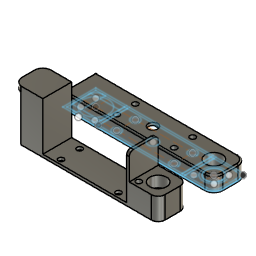
laserHolder v8 (Autodesk Fusion 360 design; units mm, degrees)
Autodesk Fusion 360 part; units mm, degrees
note: some values were not read from the file. Set by a fixed rule: which sketch regions a step uses.
sketch "Sketch1" plane through (0, 0, 0) normal (0, 0, 1) x (1, 0, 0)
  line L0 (0, 0) -> (61, 0)
  line L1 (61, 0) -> (61, 21)
  line L2 (61, 21) -> (0, 21)
  line L3 (0, 21) -> (0, 0)
  line L4 (61, 0) -> (63, 0)
  line L5 (63, 0) -> (63, 21)
  line L6 (63, 21) -> (61, 21)
  line L7 (61, 21) -> (61, 0)
  line L8 (0, 21) -> (-2, 21)
  line L9 (-2, 21) -> (-2, 0)
  line L10 (-2, 0) -> (0, 0)
  line L11 (0, 0) -> (0, 21)
  line L12 (-2, 21) -> (-23, 21)
  line L13 (-23, 21) -> (-23, 0)
  line L14 (-23, 0) -> (-2, 0)
  line L15 (-2, 0) -> (-2, 21)
  line L16 (-12.5, 21) -> (-12.5, -1.4858) construction
  line L17 (-23, 10.5) -> (-2, 10.5) construction
  circle A0 centre (-12.5, 10.5) radius 9.2
  line L18 (-23, 21) -> (-16, 21)
  line L19 (-16, 21) -> (-16, 0)
  line L20 (-16, 0) -> (-23, 0)
  line L21 (-23, 0) -> (-23, 21)
  line L22 (63, 21) -> (79, 21)
  line L23 (84, 16) -> (84, 5)
  line L24 (79, 0) -> (63, 0)
  line L25 (63, 0) -> (63, 21)
  line L26 (73.5, 21) -> (73.5, 0) construction
  line L27 (63, 10.5) -> (84, 10.5) construction
  circle A1 centre (73.5, 10.5) radius 5
  circle A2 centre (73.5, 10.5) radius 6.1
  arc A3 (84, 16) -> (79, 21) centre (79, 16) ccw
  arc A4 (79, 0) -> (84, 5) centre (79, 5) ccw
  circle A5 centre (-4.3879, 2.2553) radius 1.5
  circle A6 centre (66.1765, 3.7347) radius 2
  line L28 (0, 3.3) -> (61, 3.3) construction
  line L29 (0, 16.8) -> (61, 16.8) construction
  line L30 (10.02, 0) -> (10.02, 21) construction
  line L31 (51.78, 0) -> (51.78, 21) construction
  circle A7 centre (10.02, 3.3) radius 2
  circle A8 centre (51.78, 3.3) radius 2
  circle A9 centre (10.02, 16.8) radius 2
  circle A10 centre (51.78, 16.8) radius 2
  point P0 (84, 21)
  dimension "d1" = 61
  dimension "d2" = 21
  dimension "d3" = 2
  dimension "d4" = 2
  dimension "d5" = 21
  dimension "d6" = 21
  dimension "d7" = 21
  dimension "d8" = 18.4
  dimension "d9" = 7
  dimension "d10" = 21
  dimension "d11" = 21
  dimension "d12" = 21
  dimension "d13" = 10
  dimension "d14" = 12.2
  dimension "d15" = 5
  dimension "d35" = 3
  dimension "d38" = 4
  dimension "d44" = 3.3
  dimension "d45" = 9.22
  dimension "d46" = 41.76
  dimension "d47" = 13.5
  dimension "d48" = 4
  dimension "d49" = 4
  dimension "d50" = 4
  dimension "d51" = 4
  constraint horizontal L0
  constraint vertical L1
  constraint horizontal L2
  constraint vertical L3
  constraint coincident L0.start L3.end
  constraint horizontal L4
  constraint vertical L5
  constraint horizontal L6
  constraint vertical L7
  constraint horizontal L8
  constraint vertical L9
  constraint horizontal L10
  constraint vertical L11
  constraint horizontal L12
  constraint vertical L13
  constraint horizontal L14
  constraint vertical L15
  constraint midpoint L12 L16.start
  constraint perpendicular L14 L16
  constraint midpoint L13 L17.start
  constraint midpoint L9 L17.end
  constraint midpoint L17 A0.centre
  constraint horizontal L18
  constraint vertical L19
  constraint horizontal L20
  constraint vertical L21
  constraint horizontal L22
  constraint vertical L23
  constraint horizontal L24
  constraint vertical L25
  constraint midpoint L25 L27.start
  constraint midpoint L26 A1.centre
  constraint concentric A1 A2
  constraint coincident L22 L26.start
  constraint coincident L23 L27.end
  constraint coincident P0 L22
  constraint coincident P0 L23
  constraint tangent L22 A3
  constraint tangent L23 A3
  constraint coincident L24 L26.end
  constraint tangent L23 A4
  constraint tangent L24 A4
  constraint equal A3 A4
  constraint coincident L3 L28.start
  constraint perpendicular L3 L28
  constraint coincident L1 L28.end
  constraint coincident L3 L29.start
  constraint perpendicular L3 L29
  constraint coincident L7 L29.end
  constraint coincident L0 L30.start
  constraint coincident L2 L30.end
  constraint perpendicular L2 L30
  constraint coincident L0 L31.start
  constraint coincident L2 L31.end
  constraint perpendicular L2 L31
  constraint coincident L30 A7.centre
  constraint coincident L28 A7.centre
  constraint coincident L31 A8.centre
  constraint coincident L28 A8.centre
  constraint coincident L30 A9.centre
  constraint coincident L29 A9.centre
  constraint coincident L31 A10.centre
  constraint coincident L29 A10.centre
  measures "d1" distance of L0.start L0.end
  measures "d2" distance of L0.start L2.end
  measures "d3" distance of L0.end L4.end
  measures "d4" distance of L2.end L8.end
  measures "d5" distance of L2.end L0.start
  measures "d6" distance of L8.end L12.end
  measures "d7" distance of L8.end L9.end
  measures "d8" diameter of A0
  measures "d9" distance of L12.end L18.end
  measures "d10" distance of L12.end L13.end
  measures "d11" distance of L5.end P0
  measures "d12" distance of L5.end L4.end
  measures "d13" diameter of A1
  measures "d14" diameter of A2
  measures "d15" radius of A3
  measures "d35" diameter of A5
  measures "d38" diameter of A6
  measures "d44" distance of L0 L28
  measures "d45" distance of L1 L31
  measures "d46" distance of L30 L31
  measures "d47" distance of L28 L29
  measures "d48" diameter of A7
  measures "d49" diameter of A8
  measures "d50" diameter of A9
  measures "d51" diameter of A10
extrude "Extrude1" add sketch "Sketch1" along normal blind 2 contours L0 L1 L2 L3 L7 L11 | A7 | A8 | A9 | A10 makes body 1
extrude "Extrude2" add sketch "Sketch1" along normal blind 35 contours L3 L8 L9 L10 L11 L15 | L9 L12 L14 L15 A0 L19 | A5 bodies 1
extrude "Extrude3" add sketch "Sketch1" along normal blind 35 contours L1 L4 L5 L6 L7 L25 bodies 1
extrude "Extrude4" add sketch "Sketch1" along normal blind 16 contours L5 L22 L23 L24 L25 A3 A4 | A2 | A6 bodies 1
extrude "Extrude5" cut sketch "Sketch1" along normal blind 8 from surface at 8 contours A2 bodies 1
sketch "Sketch2" plane through (0, 0, 35) normal (0, 0, 1) x (-1, 0, 0)
  line L0 (16, -1.9918) -> (16, 0)
  line L1 (16, 0) -> (0, 0)
  line L2 (0, 0) -> (0, -21)
  line L3 (0, -21) -> (16, -21)
  line L4 (16, -21) -> (16, -19.0082)
  arc A0 (16, -1.9918) -> (16, -19.0082) centre (12.5, -10.5) ccw
  line L5 (0, 0) -> (15, 0)
  line L6 (21, -6) -> (21, -15)
  line L7 (15, -21) -> (0, -21)
  line L8 (0, -21) -> (0, 0)
  arc A1 (21, -6) -> (15, 0) centre (15, -6) ccw
  arc A2 (15, -21) -> (21, -15) centre (15, -15) ccw
  point P0 (21, 0)
  dimension "d27" = 21
  dimension "d28" = 21
  dimension "d29" = 6
  dimension "d30" = 6
  constraint horizontal L5
  constraint vertical L6
  constraint horizontal L7
  constraint vertical L8
  constraint coincident L1.end L2.start
  constraint coincident P0 L5
  constraint coincident P0 L6
  constraint tangent L5 A1
  constraint tangent L6 A1
  constraint tangent L6 A2
  constraint tangent L7 A2
  measures "d27" distance of L1.end P0
  measures "d28" distance of L1.end L2.end
  measures "d29" radius of A1
  measures "d30" radius of A2
extrude "Extrude7" add sketch "Sketch2" along normal blind 2 bodies 1
extrude "Extrude8" cut sketch "Sketch1" along normal blind 25 contours A5 bodies 1
extrude "Extrude9" cut sketch "Sketch1" along normal blind 30 contours A6 bodies 1
sketch "Sketch3" plane through (0, 0, 0) normal (0, -1, 0) x (1, 0, 0)
  line L0 (-16, 0) -> (79, 0)
  line L1 (79, 0) -> (79, 16)
  line L2 (79, 16) -> (63, 16)
  line L3 (63, 16) -> (63, 35)
  line L4 (63, 35) -> (61, 35)
  line L5 (61, 35) -> (61, 2)
  line L6 (61, 2) -> (0, 2)
  line L7 (0, 2) -> (0, 37)
  line L8 (0, 37) -> (-16, 37)
  line L9 (-16, 37) -> (-16, 0)
  line L10 (-1.7096, 20.6005) -> (-6.0859, 20.6005)
  line L11 (-6.0859, 20.6005) -> (-6.0859, 32.0028)
  line L12 (-6.0859, 32.0028) -> (-1.7096, 32.0028)
  line L13 (-1.7096, 32.0028) -> (-1.7096, 20.6005)
  constraint horizontal L10
  constraint vertical L11
  constraint horizontal L12
  constraint vertical L13
extrude "Extrude10" cut sketch "Sketch3" against normal blind 14 from surface at -1 contours L10 L11 L12 L13 bodies 1
extrude "Extrude11" cut sketch "Sketch1" along normal blind 3 contours A7 | A8 | A9 | A10 bodies 1
fillet "Fillet1" radius 0.5 1 edges at (-4.3879, 3.7553, 20.6005) on bodies 1
extrude "Extrude12" add sketch "Sketch2" against normal blind 2 contours L0 L4 A0 L6 A1 A2 bodies 1
sketch "Sketch4" plane through (0, 0, 33) normal (0, 0, -1) x (1, 0, 0)
  arc A0 (-16, -0.0839) -> (-21, -6) centre (-15, -6) ccw
  line L0 (-21, -6) -> (-21, -15)
  arc A1 (-21, -15) -> (-16, -20.9161) centre (-15, -15) ccw
  line L1 (-16, -20.9161) -> (-16, -19.0082)
  arc A2 (-16, -19.0082) -> (-16, -1.9918) centre (-12.5, -10.5) ccw
  line L2 (-16, -1.9918) -> (-16, -0.0839)
  line L3 (-21, -10.5) -> (-3.3, -10.5) construction
  line L4 (-2.6492, -14) -> (-39.3508, -14)
  line L5 (-39.3508, -14) -> (-39.3508, -7)
  line L6 (-39.3508, -7) -> (-2.6492, -7)
  line L7 (-2.6492, -7) -> (-2.6492, -14)
  line L8 (-2.6492, -14) -> (-39.3508, -7) construction
  line L9 (-39.3508, -14) -> (-2.6492, -7) construction
  line L10 (-2.1646, -4) -> (-39.8354, -4)
  line L11 (-39.8354, -4) -> (-39.8354, -17)
  line L12 (-39.8354, -17) -> (-2.1646, -17)
  line L13 (-2.1646, -17) -> (-2.1646, -4)
  line L14 (-2.1646, -4) -> (-39.8354, -17) construction
  line L15 (-39.8354, -4) -> (-2.1646, -17) construction
  point P0 (-21, -10.5)
  point P1 (-21, -10.5)
  dimension "d59" = 7
  dimension "d70" = 13
  constraint midpoint L0 P1
  constraint perpendicular L0 L3
  constraint horizontal L4
  constraint perpendicular L4 L5
  constraint parallel L4 L6
  constraint parallel L5 L7
  constraint coincident L8 P1
  constraint coincident L9 P1
  constraint coincident P1 P0
  constraint horizontal L10
  constraint perpendicular L10 L11
  constraint parallel L10 L12
  constraint parallel L11 L13
  constraint coincident L14 P1
  constraint coincident L15 P1
  measures "d59" distance of L4.end L5.end
  measures "d70" distance of L10.end L11.end
extrude "Extrude23" cut sketch "Sketch4" against normal blind 1.5 contours A0 L0 A2 L6 L10 | L0 A2 L4 L6 | L0 A1 A2 L4 L12 bodies 1
fillet "Fillet4" radius 3 1 edges at (62, 21, 35) on bodies 1
fillet "Fillet5" radius 3 1 edges at (62, 0, 35) on bodies 1
extrude "Extrude14" add sketch "Sketch4" against normal blind 1.5 contours A0 A2 L2 L10 | A1 L1 A2 L12 bodies 1
sketch "Sketch5" plane through (0, 0, 0) normal (0, 0, 1) x (1, 0, 0)
  line L0 (61, 61.5595) -> (0, 61.5595)
  line L1 (0, 61.5595) -> (-2, 61.5595)
  line L2 (10.02, 40.5595) -> (10.02, 61.5595) construction
  arc A0 (84, 56.5595) -> (79, 61.5595) centre (79, 56.5595) ccw
  line L3 (-23, 40.5595) -> (-23, 61.5595)
  line L4 (84, 56.5595) -> (84, 45.5595)
  circle A1 centre (51.78, 57.3595) radius 2
  line L5 (-2, 40.5595) -> (-2, 61.5595)
  line L6 (63, 51.0595) -> (84, 51.0595) construction
  line L7 (-23, 56.5595) -> (-23, 45.5595)
  line L8 (-23, 51.0595) -> (-2, 51.0595) construction
  circle A2 centre (66.1765, 43.7347) radius 2
  line L9 (-18, 61.5595) -> (-16, 61.5595)
  line L10 (-2, 61.5595) -> (-23, 61.5595)
  circle A3 centre (-12.5, 51.0595) radius 9.2
  line L11 (63, 40.5595) -> (63, 61.5595)
  circle A4 centre (10.02, 57.3595) radius 2
  line L12 (63, 40.5595) -> (63, 61.5595)
  line L13 (-2, 61.5595) -> (-2, 40.5595)
  line L14 (79, 40.5595) -> (63, 40.5595)
  line L15 (0, 61.5595) -> (0, 40.5595)
  line L16 (-2, 40.5595) -> (0, 40.5595)
  line L17 (0, 40.5595) -> (0, 61.5595)
  line L18 (0, 43.8595) -> (61, 43.8595) construction
  line L19 (0, 40.5595) -> (61, 40.5595)
  line L20 (0, 57.3595) -> (61, 57.3595) construction
  arc A5 (79, 40.5595) -> (84, 45.5595) centre (79, 45.5595) ccw
  line L21 (51.78, 40.5595) -> (51.78, 61.5595) construction
  line L22 (-23, 40.5595) -> (-2, 40.5595)
  line L23 (-12.5, 61.5595) -> (-12.5, 38.5142) construction
  line L24 (61, 61.5595) -> (61, 40.5595)
  line L25 (61, 40.5595) -> (63, 40.5595)
  line L26 (73.5, 61.5595) -> (73.5, 40.5595) construction
  circle A6 centre (51.78, 43.8595) radius 2
  line L27 (63, 61.5595) -> (61, 61.5595)
  line L28 (63, 61.5595) -> (79, 61.5595)
  circle A7 centre (73.5, 51.0595) radius 6
  circle A8 centre (-4.3879, 42.2553) radius 1.5
  line L29 (-16, 40.5595) -> (-18, 40.5595)
  circle A9 centre (10.02, 43.8595) radius 2
  line L30 (61, 40.5595) -> (61, 61.5595)
  circle A10 centre (73.5, 51.0595) radius 6.1
  line L31 (-16, 61.5595) -> (-16, 40.5595)
  arc A11 (-18, 61.5595) -> (-23, 56.5595) centre (-18, 56.5595) ccw
  arc A12 (-23, 45.5595) -> (-18, 40.5595) centre (-18, 45.5595) ccw
  line L32 (61, 63.0595) -> (0, 63.0595)
  line L33 (0, 63.0595) -> (-2, 63.0595)
  line L34 (-2, 63.0595) -> (-24.5, 63.0595)
  line L35 (-24.5, 39.0595) -> (-24.5, 63.0595)
  line L36 (-24.5, 39.0595) -> (-2, 39.0595)
  line L37 (-2, 39.0595) -> (0, 39.0595)
  line L38 (0, 39.0595) -> (61, 39.0595)
  line L39 (61, 39.0595) -> (63, 39.0595)
  line L40 (79, 39.0595) -> (63, 39.0595)
  arc A13 (79, 39.0595) -> (85.5, 45.5595) centre (79, 45.5595) ccw
  line L41 (85.5, 56.5595) -> (85.5, 45.5595)
  arc A14 (85.5, 56.5595) -> (79, 63.0595) centre (79, 56.5595) ccw
  line L42 (63, 63.0595) -> (79, 63.0595)
  line L43 (63, 63.0595) -> (61, 63.0595)
  circle A15 centre (51.78, 43.8595) radius 3
  circle A16 centre (10.02, 43.8595) radius 3
  circle A17 centre (10.02, 57.3595) radius 3
  circle A18 centre (51.78, 57.3595) radius 3
  circle A19 centre (73.5, 51.0595) radius 7.6
  circle A20 centre (30.5, 49.7205) radius 3.5
  line L44 (-23, 57.8325) -> (-2, 57.8325)
  line L45 (-2, 44.3325) -> (-23, 44.3325)
  point P0 (0, 40.5595)
  point P1 (84, 61.5595)
  dimension "d73" = 61
  dimension "d74" = 21
  dimension "d75" = 2
  dimension "d76" = 2
  dimension "d77" = 21
  dimension "d78" = 21
  dimension "d79" = 21
  dimension "d80" = 18.4
  dimension "d81" = 7
  dimension "d82" = 21
  dimension "d83" = 21
  dimension "d84" = 21
  dimension "d85" = 12
  dimension "d86" = 12.2
  dimension "d87" = 5
  dimension "d88" = 3
  dimension "d89" = 4
  dimension "d90" = 3.3
  dimension "d91" = 9.22
  dimension "d92" = 41.76
  dimension "d93" = 13.5
  dimension "d94" = 4
  dimension "d95" = 4
  dimension "d96" = 4
  dimension "d97" = 4
  dimension "d98" = 5
  dimension "d99" = 5
  dimension "d100" = -1.5
  dimension "d105" = 1
  dimension "d106" = 1
  dimension "d107" = 1
  dimension "d108" = 1
  dimension "d121" = 1.5
  dimension "d124" = 7
  dimension "d129" = 13.5
  constraint horizontal L19
  constraint vertical L30
  constraint horizontal L0
  constraint vertical L15
  constraint coincident P0 L15.end
  constraint horizontal L25
  constraint vertical L12
  constraint horizontal L27
  constraint vertical L24
  constraint horizontal L1
  constraint vertical L13
  constraint horizontal L16
  constraint vertical L17
  constraint horizontal L10
  constraint vertical L7
  constraint horizontal L22
  constraint vertical L5
  constraint midpoint L23.start L10
  constraint perpendicular L22 L23
  constraint midpoint L8.end L13
  constraint midpoint A3.centre L8
  constraint horizontal L9
  constraint vertical L31
  constraint horizontal L29
  constraint vertical L3
  constraint horizontal L28
  constraint vertical L4
  constraint horizontal L14
  constraint vertical L11
  constraint midpoint L6.start L11
  constraint midpoint A7.centre L26
  constraint concentric A7 A10
  constraint coincident L26.start L28
  constraint coincident L6.end L4
  constraint coincident P1 L28
  constraint coincident P1 L4
  constraint tangent A0 L28
  constraint tangent A0 L4
  constraint coincident L26.end L14
  constraint tangent L4 A5
  constraint tangent L14 A5
  constraint equal A0 A5
  constraint coincident L18.start L15
  constraint perpendicular L15 L18
  constraint coincident L18.end L30
  constraint coincident L20.start L15
  constraint perpendicular L15 L20
  constraint coincident L20.end L24
  constraint coincident L2.start L19
  constraint coincident L2.end L0
  constraint perpendicular L0 L2
  constraint coincident L21.start L19
  constraint coincident L21.end L0
  constraint perpendicular L0 L21
  constraint coincident A9.centre L2
  constraint coincident A9.centre L18
  constraint coincident A6.centre L21
  constraint coincident A6.centre L18
  constraint coincident A4.centre L2
  constraint coincident A4.centre L20
  constraint coincident A1.centre L21
  constraint coincident A1.centre L20
  constraint coincident L8.start L7
  constraint coincident L3.end L9
  constraint coincident L3.end L7
  constraint tangent L9 A11
  constraint tangent L7 A11
  constraint coincident L3.start L29
  constraint coincident L3.start L7
  constraint tangent L29 A12
  constraint tangent L7 A12
  constraint coincident L3 L44.start
  constraint perpendicular L3 L44
  constraint coincident L13 L44.end
  constraint coincident L13 L45.start
  constraint perpendicular L13 L45
  constraint coincident L3 L45.end
  measures "d73" distance of L19.end P0
  measures "d74" distance of L0.end P0
  measures "d75" distance of L11.start L19.end
  measures "d76" distance of L1.end L0.end
  measures "d77" distance of P0 L0.end
  measures "d78" distance of L1.end L3.end
  measures "d79" distance of L1.end L5.start
  measures "d80" diameter of A3
  measures "d81" distance of L9.end L3.end
  measures "d82" distance of L3.start L3.end
  measures "d83" distance of L11.end P1
  measures "d84" distance of L11.end L11.start
  measures "d85" diameter of A7
  measures "d86" diameter of A10
  measures "d87" radius of A0
  measures "d88" diameter of A8
  measures "d89" diameter of A2
  measures "d90" distance of L18 L19
  measures "d91" distance of L21 L30
  measures "d92" distance of L2 L21
  measures "d93" distance of L18 L20
  measures "d94" diameter of A9
  measures "d95" diameter of A6
  measures "d96" diameter of A4
  measures "d97" diameter of A1
  measures "d98" radius of A11
  measures "d99" radius of A12
  measures "d124" diameter of A20
  measures "d129" distance of L44 L45
extrude "Extrude15" add sketch "Sketch5" along normal blind 11 from surface at -1 separate body contours L32 L33 L34 L35 L36 L37 L38 L39 L40 A13 L41 A14 L42 L43 makes body 2
extrude "Extrude18" add sketch "Sketch5" along normal blind 2 from surface at 8 separate body contours L0 L15 L17 L19 L24 L30 | L11 L12 L24 L25 L27 L30 | L1 L5 L13 L15 L16 L17 | A0 L4 L11 L12 L14 A5 L28 | L5 L10 A3 L13 L31 L44 | L5 A3 L13 L44 L45 | L9 L10 A3 L31 A11 L44 | L5 A3 L13 L22 L31 L45 | A3 L31 L44 | A3 L31 L44 L45 | L3 L10 A11 L44 | A3 L31 L44 | A3 L22 L29 L31 A12 L45 | A3 L31 L45 | A3 L31 L44 L45 | L3 L7 A3 A11 A12 L44 L45 | L3 A11 L44 | L3 L22 A12 L45 | A3 L31 L45 | L3 A12 L45 | A2 | A8 | A19 | A20 makes body 3
fillet "Fillet7" radius 1 5 edges at (27.25, 39.0595, 10) (83.5962, 40.9633, 10) (85.5, 51.0595, 10) (83.5962, 61.1556, 10) (27.25, 63.0595, 10) on bodies 2
fillet "Fillet8" radius 1 5 edges at (-24.5, 63.0595, 4) (-24.5, 62.7666, 9.7071) (-24.5, 51.0595, 10) (-24.5, 39.3523, 9.7071) (-24.5, 39.0595, 4) on bodies 2
extrude "Extrude19" add sketch "Sketch5" along normal blind 10 contours A19 bodies 3
extrude "Extrude20" cut sketch "Sketch5" along normal blind 30 contours A20 bodies 3
extrude "Extrude21" add sketch "Sketch5" against normal blind 1 from surface at 8 contours L5 A3 L13 L22 L31 L45 | A3 L22 L29 L31 A12 L45 | A3 L31 L45 | A3 L31 L45 | A8 bodies 2 3
extrude "Extrude22" add sketch "Sketch5" against normal blind 1 from surface at 8 contours L5 L10 A3 L13 L31 L44 | L9 L10 A3 L31 A11 L44 | A3 L31 L44 | A3 L31 L44 bodies 2
extrude "Extrude24" add sketch "Sketch5" along normal blind 9 from surface at 1 contours A15 | A16 | A17 | A18 bodies 2
